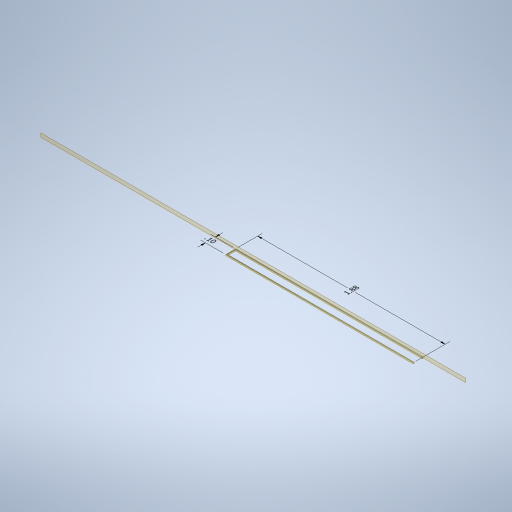
# Autodesk Inventor part: basic strain gauge 0p01 long
Saved by Autodesk Inventor 2024.2 (Build 282272000, 272)
## iProperties
Created: 2024-07-17
Part Number: basic strain gauge 0p01 long
Material: Silver
Document SubType Name: Modeling
Designer: Makerspace
Density: 10.49 g/cm^3
Appearance: Silver
Author: Makerspace
Autodesk Inventor part; units mm, degrees
ref_plane "XZ Plane" through (0, 0, 0) normal (0, 1, 0) x (-1, 0, 0)
sketch "Sketch1" plane through (0, 0, 0) normal (0, 1, 0) x (-1, 0, 0)
  line L0 (0, 0) -> (47.625, 0)
  line L1 (47.625, -2.54) -> (0, -2.54)
  line L2 (47.625, -2.54) -> (47.625, 0)
  dimension "d69" = 47.625
  dimension "d70" = 47.625
  dimension "d89" = 2.54
  dimension "d90" = 0
  dimension "d91" = 0
  dimension "d92" = 0
  constraints: 6 end point, 1 horizontal, 1 vertical
  measures "d69" distance of L1.start L1.end
  measures "d70" distance of L0.start L0.end
  measures "d89" distance of L1.start L0.end
  measures "d90" distance of point (0, 0) L0.start
  measures "d91" horizontal distance of point (0, 0) L1.end
  measures "d92" distance of point (0, 0) L0.start
sketch "Sketch2" plane through (0, 0, 0) normal (1, 0, 0) x (0, 1, 0)
  line L0 (0, 0) -> (0.254, 0)
  line L1 (0.254, 0) -> (0.254, -0.254)
  line L2 (0.254, -0.254) -> (0, -0.254)
  line L3 (0, -0.254) -> (0, 0)
  dimension "d98" = 0.254
  dimension "d99" = 0.254
  constraints: 8 end point, 2 parallel, 1 horizontal, 1 perpendicular
  measures "d98" distance of L0.end L1.end
  measures "d99" distance of L1.end L2.end
sweep "Sweep1" add profiles "Sketch2" path "Sketch1"
ref_plane "Work Plane1" through (6.35, 0, 0) normal (1, 0, 0) x (0, 1, 0)
ref_plane "Work Plane2" through (0, 0, -6.35) normal (0, 0, 1) x (1, 0, 0)
ref_plane "Work Plane4" through (0, 0, -2.9845) normal (0, 0, 1) x (1, 0, 0)
body "Solid1"
